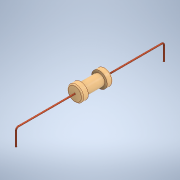
# Autodesk Inventor part: МЛТ-1
Saved by Autodesk Inventor 2020.2 (Build 242310000, 310)
## iProperties
Created: 2020-03-30
Part Number: МЛТ-1
Material: Copper
Document SubType Name: Modeling
Designer: IAmIllusion
Density: 8.94 g/cm^3
Appearance: Copper - Satin
Author: IAmIllusion
Autodesk Inventor part; units mm, degrees
ref_plane "YZ Plane" through (0, 0, 0) normal (1, 0, 0) x (0, 1, 0)
ref_plane "XZ Plane" through (0, 0, 0) normal (0, 1, 0) x (-1, 0, 0)
ref_plane "XY Plane" through (0, 0, 0) normal (0, 0, 1) x (1, 0, 0)
sketch "Sketch1" plane through (0, 0, 0) normal (1, 0, 0) x (0, 1, 0)
  line L0 (0.5, 0) -> (6.1, 0)
  line L1 (6.6, 0.5) -> (6.6, 2.5)
  line L2 (6.6, 2.5) -> (5.6, 2.5)
  line L3 (5.6, 2.5) -> (5.6, 10.5)
  line L4 (5.6, 10.5) -> (6.6, 10.5)
  line L5 (6.6, 10.5) -> (6.6, 12.5)
  line L6 (6.1, 13) -> (0.5, 13)
  line L7 (0, 12.5) -> (0, 10.5)
  line L8 (0, 10.5) -> (1, 10.5)
  line L9 (1, 10.5) -> (1, 2.5)
  line L10 (1, 2.5) -> (0, 2.5)
  line L11 (0, 2.5) -> (0, 0.5)
  arc A0 (6.6, 12.5) -> (6.1, 13) centre (6.1, 12.5) ccw
  arc A1 (0.5, 13) -> (0, 12.5) centre (0.5, 12.5) ccw
  arc A2 (6.1, 0) -> (6.6, 0.5) centre (6.1, 0.5) ccw
  arc A3 (0, 0.5) -> (0.5, 0) centre (0.5, 0.5) ccw
  line L12 (3.3, 13) -> (3.3, 0)
  point P0 (6.6, 13)
  constraints: 26 end point, 8 point on circle, 8 point on line, 8 tangent, 5 perpendicular, 4 centre point, 2 midpoint, 1 equal radius, 1 horizontal
sketch "Sketch2" plane through (0, 0, 0) normal (1, 0, 0) x (0, 1, 0)
  line L0 (3.3, 13) -> (3.3, 37)
  line L1 (2.3, 38) -> (-3.7, 38)
  arc A0 (3.3, 37) -> (2.3, 38) centre (2.3, 37) ccw
  constraints: 4 end point, 2 point on circle, 2 tangent, 1 centre point, 1 horizontal, 1 vertical
sketch "Sketch3" plane through (0, 0, 0) normal (1, 0, 0) x (0, 1, 0)
  line L0 (3.3, 0) -> (3.3, -24)
  line L1 (2.3, -25) -> (-3.7, -25)
  arc A0 (2.3, -25) -> (3.3, -24) centre (2.3, -24) ccw
  constraints: 4 end point, 2 point on circle, 2 tangent, 1 centre point, 1 horizontal, 1 vertical
sketch "Sketch4" plane through (0, 0, 0) normal (0, 1, 0) x (-1, 0, 0)
  circle A0 centre (0, 38.0001) radius 0.3
  point P0 (0, 0)
  constraints: 1 centre point
sketch "Sketch5" plane through (0, 0, 0) normal (0, 1, 0) x (-1, 0, 0)
  circle A0 centre (0, -24.9999) radius 0.3
  point P0 (0, 0)
  constraints: 1 centre point
sweep "Sweep1" add profiles "Sketch4" path "Sketch2"
sweep "Sweep2" add profiles "Sketch5" path "Sketch3" separate body
revolve "Revolution2" add sketch "Sketch1" angle 360 about axis through (0, 3.3, 13) along (0, 0, -1) bodies 1 contours L12 L6 A0 L5 L4 L3 L2 L1 A2 L0
body "Solid1"
body "Solid2"
body "Solid3"
